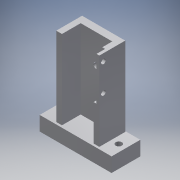
# Autodesk Inventor part: XPulleySupportBase
Saved by Autodesk Inventor 2019 (Build 230136000, 136)
## iProperties
Created: 2019-08-19
Part Number: XPulleySupportBase
Material: ABS Plastic
Document SubType Name: Modeling
Designer: Bruno
Density: 1.06 g/cm^3
Appearance: Smooth - White
Mass: 21.3055 g
Surface Area: 92.1532 cm^2
Volume: 20.0995 cm^3
Author: Bruno
## iProperties of the stored document XPulleySupportBase_3DPrint.ipt
Created: 2019-09-09
Part Number: XPulleySupportBase_3DPrint
Material: Generic
Document SubType Name: Modeling
Designer: Bruno
Density: 1 g/cm^3
Appearance: Default
Author: Bruno
Autodesk Inventor part; units mm, degrees
ref_plane "YZ Plane" through (0, 0, 0) normal (1, 0, 0) x (0, 1, 0)
ref_plane "XZ Plane" through (0, 0, 0) normal (0, 1, 0) x (-1, 0, 0)
ref_plane "XY Plane" through (0, 0, 0) normal (0, 0, 1) x (1, 0, 0)
sketch "Sketch2" plane through (0, 0, 0) normal (0, 1, 0) x (-1, 0, 0)
  line L0 (10.6557, -7.541) -> (-39.3443, -7.541)
  line L1 (-39.3443, -7.541) -> (-39.3443, 12.459)
  line L2 (-39.3443, 12.459) -> (10.6557, 12.459)
  line L3 (10.6557, 12.459) -> (10.6557, -7.541)
  point P0 (0, 0)
  dimension "d10" = 20
  dimension "d11" = 50
  constraints: 8 end point, 2 parallel, 1 horizontal, 1 perpendicular
  measures "d10" distance of L2.end L0.start
  measures "d11" distance of L0.start L0.end
extrude "Extrusion3" add sketch "Sketch2" along normal blind 10
sketch "Sketch3" plane through (0, 10, 0) normal (0, 1, 0) x (1, 0, 0)
  line L0 (39.3443, 7.541) -> (-10.6557, 7.541) projected
  line L1 (-10.6557, 7.541) -> (-10.6557, -12.459) projected
  line L2 (-10.6557, -12.459) -> (39.3443, -12.459) projected
  line L3 (39.3443, -12.459) -> (39.3443, 7.541) projected
  line L4 (-1.6557, -10.959) -> (-1.6557, 7.041)
  line L5 (-1.6557, 7.041) -> (30.3443, 7.041)
  line L6 (30.3443, 7.041) -> (30.3443, -10.959)
  line L7 (30.3443, -10.959) -> (25.3443, -10.959)
  line L8 (25.3443, -10.959) -> (25.3443, 2.041)
  line L9 (25.3443, 2.041) -> (3.3443, 2.041)
  line L10 (3.3443, 2.041) -> (3.3443, -10.959)
  line L11 (3.3443, -10.959) -> (-1.6557, -10.959)
  line L12 (-1.6557, 7.041) -> (-10.6557, 7.041) construction
  line L13 (30.3443, 7.041) -> (39.3443, 7.041) construction
  line L14 (-1.6557, 7.041) -> (-1.6557, 7.541) construction
  point P0 (0, 0)
  dimension "d14" = 22
  dimension "d15" = 5
  dimension "d16" = 5
  dimension "d17" = 0.5
  dimension "d18" = 13
  constraints: 22 end point, 9 perpendicular, 5 point on line, 2 collinear, 1 vertical
  measures "d14" distance of L8.end L9.end
  measures "d15" distance of L6.end L7.end
  measures "d16" distance between parallel lines of L5 L9
  measures "d17" distance of L4.end L14.end
  measures "d18" distance of L9.end L10.end
extrude "Extrusion4" add sketch "Sketch3" along normal blind 55 contours L4 L5 L6 L7 L8 L9 L10 L11
sketch "Sketch4" plane through (30.3443, 10, -7.041) normal (0, 0, -1) x (-1, 0, 0)
  circle A0 centre (16, 34.875) radius 2.125
  line L0 (16, 34.875) -> (0, 34.875) construction
  line L1 (0, 0) -> (0, 55) projected
  line L2 (16, 34.875) -> (32, 34.875) construction
  line L3 (32, 0) -> (32, 55) projected
  line L4 (0, 55) -> (32, 55) projected
  line L5 (-9, 0) -> (41, 0) projected
  point P0 (30.3443, -10)
  point P1 (28, 0)
  dimension "d21" = 4.25
  dimension "d32" = 34.875
  constraints: 4 end point, 2 point on line, 1 centre point, 1 collinear, 1 horizontal, 2 other
  measures "d21" diameter of A0
  measures "d32" distance between parallel lines of L0 L5
extrude "Extrusion5" cut sketch "Sketch4" against normal up to next contours A0
sketch "Sketch5" plane through (0, 10, 0) normal (0, 1, 0) x (1, 0, 0)
  circle A0 centre (-5.6557, -2.459) radius 2.125
  circle A1 centre (34.3443, -2.459) radius 2.125
  line L0 (-5.6557, -2.459) -> (-10.6557, -2.459) construction
  line L1 (34.3443, -2.459) -> (39.3443, -2.459) construction
  line L2 (39.3443, -12.459) -> (39.3443, 7.541) projected
  line L3 (39.3443, 7.541) -> (-10.6557, 7.541) projected
  line L4 (-10.6557, 7.541) -> (-10.6557, -12.459) projected
  point P0 (0, 0)
  dimension "d26" = 4.25
  dimension "d27" = 10
  dimension "d28" = 5
  constraints: 4 end point, 2 centre point, 2 collinear, 2 horizontal, 2 midpoint, 1 equal radius
  measures "d26" diameter of A0
  measures "d27" distance between parallel lines of L3 L0
  measures "d28" distance of L0.start L0.end
extrude "Extrusion6" cut sketch "Sketch5" against normal up to next
sketch "Sketch6" plane through (30.3443, 10, 10.959) normal (1, 0, 0) x (0, 0, -1)
  circle A0 centre (2.8, 31) radius 1.625
  circle A1 centre (2.8, 50) radius 1.625
  line L0 (18, 0) -> (0, 0) projected
  line L1 (0, 0) -> (0, 55) projected
  line L2 (2.8, 50) -> (2.8, 31) construction
  point P0 (10.959, -10)
  dimension "d33" = 3.25
  dimension "d34" = 3.25
  dimension "d35" = 19
  dimension "d36" = 31
  dimension "d37" = 2.8
  constraints: 2 centre point, 2 end point, 1 vertical
  measures "d33" diameter of A0
  measures "d34" diameter of A1
  measures "d35" distance of L2.end L2.start
  measures "d36" distance from line of L2.end L0
  measures "d37" distance from line of L1 L2.end
extrude "Extrusion7" cut sketch "Sketch6" against normal up to surface (5 mm away)
sketch "Sketch7" plane through (25.3443, 10, -2.041) normal (-1, 0, 0) x (0, 0, 1)
  line L0 (0, 55) -> (13, 55) projected
  line L1 (7, 55) -> (7, 25)
  line L2 (7, 25) -> (13, 25)
  line L3 (13, 0) -> (13, 55) projected
  line L4 (13, 25) -> (13, 55)
  line L5 (7, 55) -> (13, 55)
  point P0 (2.041, -10)
  dimension "d40" = 6
  dimension "d41" = 30
  constraints: 8 end point, 2 collinear, 1 horizontal, 1 perpendicular, 1 point on line, 1 vertical
  measures "d40" distance between parallel lines of L3 L1
  measures "d41" distance of L1.start L1.end
extrude "Extrusion8" cut sketch "Sketch7" against normal blind 2
body "Solid2"
